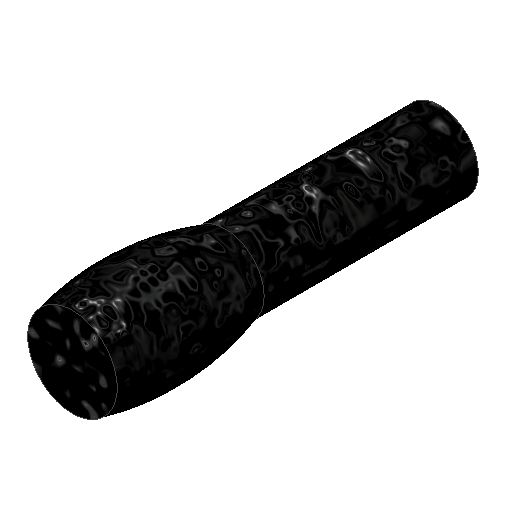
# Autodesk Inventor part: 00_flashlight_FX_light_FC4_Pollin
Saved by Autodesk Inventor 2022 (Build 260153000, 153)
## iProperties
Created: 2020-12-04
Part Number: 00_flashlight_FX_light_FC4_Pollin
Material: Generic
Document SubType Name: Modeling
Designer: UC2
Density: 1 g/cm^3
Appearance: Schwarz
Catalog Web Link: https://www.pollin.de/p/daylite-led-taschenlampe-my-75171-mblack-schwarz-535804
Vendor: Aliexpress
Author: UC2
Autodesk Inventor part; units mm, degrees
ref_plane "YZ Plane" through (0, 0, 0) normal (1, 0, 0) x (0, 1, 0)
ref_plane "XZ Plane" through (0, 0, 0) normal (0, 1, 0) x (-1, 0, 0)
ref_plane "XY Plane" through (0, 0, 0) normal (0, 0, 1) x (1, 0, 0)
sketch "Skizze1" plane through (0, 0, 0) normal (0, 0, 1) x (1, 0, 0)
  circle A0 centre (0, 0) radius 13.95
  dimension "d0" = 27.9
  constraints: 1 centre point, 1 coincident
  measures "d0" diameter of A0
extrude "Extrusion1" add sketch "Skizze1" along normal blind 77
sketch "Skizze2" plane through (0, 0, 0) normal (1, 0, 0) x (0, 1, 0)
  line L0 (13.95, 0) -> (13.95, 77) projected
  arc A0 (13.95, 77) -> (16.085, 131.9585) centre (-81.6004, 108.2326) ccw
  line L1 (16.085, 131.9585) -> (0, 131.9585)
  line L2 (0, 131.9585) -> (0, 77)
  line L3 (13.95, 77) -> (-13.95, 77) projected
  line L4 (13.95, 77) -> (0, 77)
  line L5 (18.925, 132.8212) -> (18.925, 80.1833)
  point P0 (0, 0)
  dimension "d3" = 55
  dimension "d4" = 18.925
  dimension "d6" = 16.085
  constraints: 8 end point, 2 point on circle, 1 centre point, 1 horizontal, 1 midpoint, 1 perpendicular, 1 point on line, 1 tangent, 1 vertical
  measures "d3" distance of L3.start L1.start
  measures "d4" distance between parallel lines of L2 L5
  measures "d6" distance of L1.end L1.start
revolve "Umdrehung1" add sketch "Skizze2" angle 360 about axis through (0, 0, 131.9585) along (0, 0, -1)
